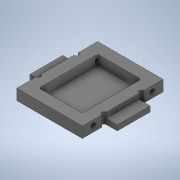
# Autodesk Inventor part: Cockpit_vertical_frame_04
Saved by Autodesk Inventor 2020.4 (Build 244396000, 396)
## iProperties
Created: 2021-04-12
Part Number: Cockpit_vertical_frame_04
Material: アセタール樹脂、黒
Document SubType Name: Modeling
Designer: Masato Kubotera
Density: 1.425 g/cm^3
Appearance: 滑らか - 黒
Mass: 7.89081 g
Surface Area: 35.2093 cm^2
Volume: 5.53741 cm^3
Author: Masato Kubotera
Title: Cockpit_vertical_frame_04
Autodesk Inventor part; units mm, degrees
ref_plane "YZ Plane" through (0, 0, 0) normal (1, 0, 0) x (0, 1, 0)
ref_plane "XZ Plane" through (0, 0, 0) normal (0, 1, 0) x (-1, 0, 0)
ref_plane "XY Plane" through (0, 0, 0) normal (0, 0, 1) x (1, 0, 0)
sketch "スケッチ2" plane through (15, 9.6, 0) normal (1, 0, 0) x (0, 0, -1)
  line L0 (0, 8.9) -> (-5, 8.9) projected
  line L1 (-2.5, 8.9) -> (-2.5, -28.1) construction
  line L2 (0, -28.1) -> (-5, -28.1) projected
  line L3 (-5, -2.1) -> (-5, -17.1) construction
  line L4 (-5, -9.6) -> (0, -9.6) construction
  line L5 (0, -17.1) -> (0, -2.1) construction
  line L6 (-2.5, -28.1) -> (-2.5, 8.9) construction
  point P0 (-2.5, 3.9)
  point P1 (-2.5, -23.1)
  dimension "d52" = 5
  constraints: 6 end point, 4 midpoint, 3 symmetric about line, 2 point on line
  measures "d52" distance from line of point (-2.5, 3.9) L0
sketch "スケッチ1" plane through (0, 0, 0) normal (0, 0, 1) x (1, 0, 0)
  line L0 (-15, 18.5) -> (-15, 9.6)
  line L1 (-20, 7.5) -> (-15, 7.5)
  line L2 (-19.5911, 0) -> (20.4089, 0) construction
  line L3 (0, 18.5) -> (0, -18.5) construction
  line L4 (-20, -7.5) -> (-15, -7.5)
  arc A0 (-15, 7.5) -> (-15, 9.6) centre (-15, 8.55) ccw
  arc A1 (-15, -9.6) -> (-15, -7.5) centre (-15, -8.55) ccw
  line L5 (-20, -7.5) -> (-20, 7.5)
  line L6 (-15, -9.6) -> (-15, -18.5)
  line L7 (-15, 18.5) -> (15, 18.5)
  line L8 (15, 18.5) -> (15, 9.6)
  line L9 (20, 7.5) -> (15, 7.5)
  line L10 (20, -7.5) -> (15, -7.5)
  arc A2 (15, 9.6) -> (15, 7.5) centre (15, 8.55) ccw
  arc A3 (15, -7.5) -> (15, -9.6) centre (15, -8.55) ccw
  line L11 (15, -9.6) -> (15, -18.5)
  line L12 (20, 7.5) -> (20, -7.5)
  line L13 (15, 7.5) -> (15, -7.5)
  line L14 (-15, 7.5) -> (-15, -7.5)
  line L15 (-15, -18.5) -> (15, -18.5)
  line L16 (-10, 13.5) -> (10, 13.5)
  line L17 (10, 13.5) -> (10, -13.5)
  line L18 (10, -13.5) -> (-10, -13.5)
  line L19 (-10, -13.5) -> (-10, 13.5)
  line L20 (-10, 13.5) -> (10, -13.5) construction
  line L21 (10, 13.5) -> (-10, -13.5) construction
  point P0 (0, 0)
  point P1 (-15, -7.5)
  dimension "d4" = 15
  dimension "d5" = 1.05
  dimension "d8" = 40
  dimension "d12" = 5
  dimension "d41" = 30
  dimension "d51" = 37
  dimension "d60" = 5
  dimension "d61" = 5
  constraints: 44 end point, 16 symmetric about line, 8 point on circle, 6 point on line, 5 perpendicular, 4 centre point, 3 midpoint, 2 horizontal, 2 parallel, 2 vertical, 1 collinear, 3 other
  measures "d4" distance between parallel lines of L4 L1
  measures "d5" radius of A0
  measures "d8" distance between parallel lines of L12 L5
  measures "d12" distance between parallel lines of L5 L0
  measures "d41" distance of L0.start L7.end
  measures "d51" distance of L15.end L7.end
  measures "d60" horizontal distance of L16.end L7.end
  measures "d61" horizontal distance of L7.end L16.end
extrude "押し出し1" add sketch "スケッチ1" along normal blind 5 contours L7 L8 A2 L13 A3 L11 L15 L6 A1 L14 A0 L0
extrude "押し出し2" add sketch "スケッチ1" along normal blind 2.5 contours L14 L4 L5 L1 | L9 L12 L10 L13
hole "穴1" at (15, 13.5, 2.5) at (15, -13.5, 2.5) direction (-1, 0, 0) diameter 2.459 depth 5 thread size "M3x0.5" class "6H" standard "ISO Metric profile"
sketch "スケッチ3" plane through (-15, 9.6, 5) normal (-1, 0, 0) x (0, 0, 1)
  arc A0 (-1.2705, 3.9) -> (-3.7295, 3.9) centre (-2.5, 3.9) ccw projected
  arc A1 (-3.7295, -23.1) -> (-1.2705, -23.1) centre (-2.5, -23.1) ccw projected
  point P0 (-5, -9.6)
  point P1 (-2.5, 3.9)
  point P2 (-2.5, -23.1)
  point P3 (-2.5, 2.6705)
  point P4 (-2.5, -21.8705)
  constraints: 2 coincident
hole "穴2" at (-15, 13.5, 2.5) at (-15, -13.5, 2.5) direction (1, 0, 0) diameter 2.459 depth 5 thread size "M3x0.5" class "6H" standard "ISO Metric profile"
extrude "押し出し3" add sketch "スケッチ1" along normal blind 0.5 contours L16 L17 L18 L19
fillet "フィレット2" radius 1 8 edges at (-10, -13.5, 0.8852) (-10, -13.5, 4.3647) (-10, 13.5, 0.8852) (-10, 13.5, 4.3647) (10, 13.5, 0.8852) (10, 13.5, 4.3647) (10, -13.5, 0.8852) (10, -13.5, 4.3647)
equation "\"d61\" = d60"
